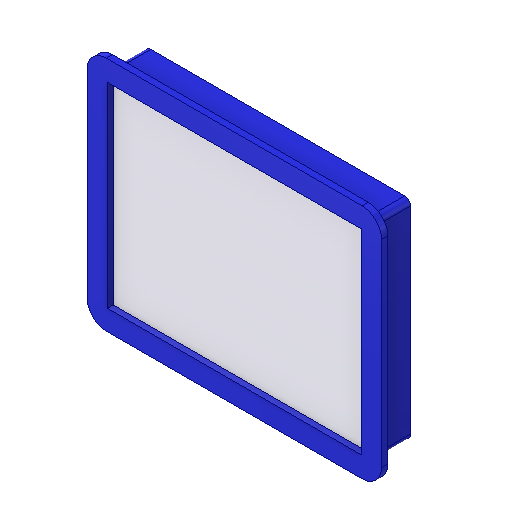
# Autodesk Inventor part: COTS_Zelmer_108x137mm_HEPA_filter
Saved by Autodesk Inventor 2026.1 (Build 301233000, 233)
## iProperties
Created: 2020-03-28
Part Number: COTS_Zelmer_108x137mm_HEPA_filter
Material: Generic
Document SubType Name: Modeling
Designer: Andrzej
Density: 1 g/cm^3
Appearance: Blue - Wall Paint - Glossy
Author: Andrzej
Autodesk Inventor part; units mm, degrees
ref_plane "YZ Plane" through (0, 0, 0) normal (1, 0, 0) x (0, 1, 0)
ref_plane "XZ Plane" through (0, 0, 0) normal (0, 1, 0) x (-1, 0, 0)
ref_plane "XY Plane" through (0, 0, 0) normal (0, 0, 1) x (1, 0, 0)
sketch "Sketch1" plane through (0, 0, 0) normal (0, 0, 1) x (1, 0, 0)
  line L0 (-66.4589, 47.2807) -> (70.5411, 47.2807)
  line L1 (70.5411, 47.2807) -> (70.5411, -60.7193)
  line L2 (70.5411, -60.7193) -> (-66.4589, -60.7193)
  line L3 (-66.4589, -60.7193) -> (-66.4589, 47.2807)
  line L4 (68.9411, 45.6807) -> (-64.8589, 45.6807)
  line L5 (-64.8589, 45.6807) -> (-64.8589, -59.1193)
  line L6 (-64.8589, -59.1193) -> (68.9411, -59.1193)
  line L7 (68.9411, -59.1193) -> (68.9411, 45.6807)
  point P0 (0, 0)
  dimension "d0" = 137
  dimension "d1" = 108
  dimension "d2" = 1.6
  constraints: 16 end point, 4 parallel, 2 perpendicular, 1 horizontal, 3 other
  measures "d0" distance of L1.end L2.end
  measures "d1" distance of L0.end L1.end
  measures "d2" distance between parallel lines of L0 L4
extrude "Extrusion1" add sketch "Sketch1" along normal blind 19.2 contours L0 L1 L2 L3 | L7 L6 L5 L4
extrude "Extrusion2" cut sketch "Sketch1" along normal blind 6.6 contours L7 L6 L5 L4
sketch "Sketch2" plane through (0, 0, 19.2) normal (0, 0, 1) x (1, 0, 0)
  line L0 (-73.9589, 54.2807) -> (78.0411, 54.2807)
  line L1 (78.0411, 54.2807) -> (78.0411, -67.7193)
  line L2 (78.0411, -67.7193) -> (-73.9589, -67.7193)
  line L3 (-73.9589, -67.7193) -> (-73.9589, 54.2807)
  line L4 (70.5411, 47.2807) -> (-66.4589, 47.2807) projected
  line L5 (70.5411, -60.7193) -> (70.5411, 47.2807) projected
  point P0 (0, 0)
  dimension "d7" = 152
  dimension "d8" = 122
  dimension "d9" = 7
  dimension "d10" = 7.5
  constraints: 8 end point, 2 parallel, 1 horizontal, 1 perpendicular
  measures "d7" distance of L1.end L2.end
  measures "d8" distance of L0.end L1.end
  measures "d9" distance between parallel lines of L0 L4
  measures "d10" distance between parallel lines of L1 L5
extrude "Extrusion3" add sketch "Sketch2" along normal blind 3.2
fillet "Fillet1" radius 3 8 edges at (70.5411, 47.2807, 9.6) (-66.4589, 47.2807, 9.6) (70.5411, -60.7193, 9.6) (-66.4589, -60.7193, 9.6) (68.9411, 45.6807, 3.3) (-64.8589, 45.6807, 3.3) (68.9411, -59.1193, 3.3) (-64.8589, -59.1193, 3.3)
fillet "Fillet2" radius 10 4 edges at (-73.9589, 54.2807, 20.8) (-73.9589, -67.7193, 20.8) (78.0411, -67.7193, 20.8) (78.0411, 54.2807, 20.8)
sketch "Sketch3" plane through (0, 0, 22.4) normal (0, 0, 1) x (1, 0, 0)
  arc A0 (78.0411, 44.2807) -> (68.0411, 54.2807) centre (68.0411, 44.2807) ccw projected
  line L0 (68.0411, 54.2807) -> (-63.9589, 54.2807) projected
  arc A1 (-63.9589, 54.2807) -> (-73.9589, 44.2807) centre (-63.9589, 44.2807) ccw projected
  line L1 (-73.9589, 44.2807) -> (-73.9589, -57.7193) projected
  arc A2 (-73.9589, -57.7193) -> (-63.9589, -67.7193) centre (-63.9589, -57.7193) ccw projected
  line L2 (-63.9589, -67.7193) -> (68.0411, -67.7193) projected
  arc A3 (68.0411, -67.7193) -> (78.0411, -57.7193) centre (68.0411, -57.7193) ccw projected
  line L3 (78.0411, -57.7193) -> (78.0411, 44.2807) projected
  line L4 (-63.4589, 43.7807) -> (67.5411, 43.7807)
  line L5 (67.5411, 43.7807) -> (67.5411, -57.2193)
  line L6 (67.5411, -57.2193) -> (-63.4589, -57.2193)
  line L7 (-63.4589, -57.2193) -> (-63.4589, 43.7807)
  point P0 (0, 0)
  dimension "d15" = 10.5
  constraints: 8 end point, 3 other
  measures "d15" distance between parallel lines of L0 L4
extrude "Extrusion4" cut sketch "Sketch3" against normal blind 3 contours L4 L5 L6 L7
equation "\"d9\" = -0.5 * d1 + 0.5 * d8"
equation "\"d10\" = -0.5 * d0 + 0.5 * d7"
body "Solid1"
